Standard Spacing Block 90 degree_v1 (Autodesk Fusion 360 design; units mm, degrees)
Autodesk Fusion 360 part; units mm, degrees
sketch "Sketch1" plane through (0, 0, 0) normal (1, 0, 0) x (0, 1, 0)
  line L0 (0, 0) -> (63.5, 0)
  line L1 (63.5, 0) -> (63.5, 63.5)
  line L2 (63.5, 63.5) -> (0, 0)
  dimension "d1" = 63.5
  constraint coincident L0.start L2.end
  constraint horizontal L0
  constraint perpendicular L0 L1
  constraint equal L0 L1
  measures "d1" distance of L0.start L0.end
extrude "Extrude1" add sketch "Sketch1" along normal mid plane 38.1
sketch "Sketch2" plane through (0, 0, 0) normal (0, 0, -1) x (1, 0, 0)
  line L0 (-19.05, -63.5) -> (19.05, -63.5)
  line L1 (19.05, -63.5) -> (19.05, 0)
  line L2 (19.05, 0) -> (-19.05, 0)
  line L3 (-19.05, 0) -> (-19.05, -63.5)
  circle A0 centre (0.0962, -12.6996) radius 6.8134
  circle A1 centre (0, -50.8) radius 6.965
  dimension "d10" = 12.7
  dimension "d11" = 12.7
  measures "d10" distance of origin A0.centre
  measures "d11" distance of L0 A1.centre
sketch "Sketch3" plane through (0, 63.5, 0) normal (0, 1, 0) x (-1, 0, 0)
  line L0 (19.05, 63.5) -> (-19.05, 63.5)
  line L1 (-19.05, 63.5) -> (-19.05, 0)
  line L2 (-19.05, 0) -> (19.05, 0)
  line L3 (19.05, 0) -> (19.05, 63.5)
  circle A0 centre (0.3187, 25.398) radius 3.175
  circle A1 centre (0, 57.15) radius 3.175
  dimension "d12" = 25.4
  dimension "d13" = 6.35
  dimension "d14" = 6.35
  dimension "d15" = 6.35
  measures "d12" distance of origin A0.centre
  measures "d13" distance of L0 A1.centre
  measures "d14" diameter of A0
  measures "d15" diameter of A1
hole "Hole3" at (0, 63.5, 57.15) at (-0.3187, 63.5, 25.398) direction (0, -1, 0) diameter 3.175 depth 19.05 tip angle 180
hole "Hole4" at (0, 50.8, 0) at (0.0962, 12.6996, 0) direction (0, 0, 1) diameter 3.175 depth 19.05 tip angle 180
equation "d17 = ( 1 / 8 ) * 1 in"
